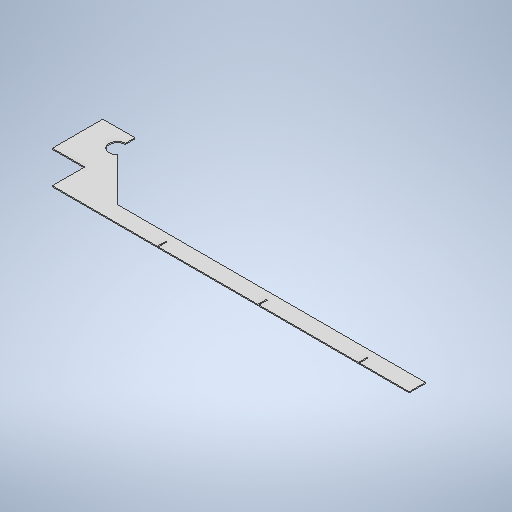
# Autodesk Inventor part: BSH 021 rib 1
Saved by Autodesk Inventor 2025 (Build 290162010, 162A)
## iProperties
Created: 2024-07-23
Part Number: BSH 021 rib 1
Material: 09g2s
Document SubType Name: Sheet Metal
Designer: admin
Density: 7.85 g/cm^3
Sheet Metal Rule: AISI304 3mm Die 32
Appearance: Default
Author: admin
Autodesk Inventor part; units mm, degrees
ref_plane "YZ Plane" through (0, 0, 0) normal (1, 0, 0) x (0, 1, 0)
ref_plane "XZ Plane" through (0, 0, 0) normal (0, 1, 0) x (-1, 0, 0)
ref_plane "XY Plane" through (0, 0, 0) normal (0, 0, 1) x (1, 0, 0)
sketch "Sketch1" plane through (0, 0, 0) normal (0, 0, 1) x (1, 0, 0)
  line L0 (1200, 2900) -> (-1200, 2900)
  line L1 (-1200, 2900) -> (-1200, 0)
  line L2 (-1200, 0) -> (1200, 0)
  line L3 (1200, 0) -> (1200, 2900)
  line L4 (1150, 2900) -> (1150, 0)
  line L5 (-1150, 0) -> (-1150, 2900) construction
  line L6 (0, 2900) -> (0, 50) construction
  line L7 (-1100, 200.463) -> (-949.537, 50)
  line L8 (-1200, 100) -> (-1100, 100)
  line L9 (-1100, 100) -> (-1100, 0)
  line L10 (-1100, 200.463) -> (-1150, 2900)
  arc A0 (-1100.463, 225.4587) -> (-1082.3223, 182.7853) centre (-1100, 200.463) ccw
  arc A1 (-1082.3223, 182.7853) -> (-1100.463, 225.4587) centre (-1100, 200.463) ccw construction
  line L11 (-1200, 255.463) -> (-1101.0187, 255.463)
  line L12 (0, 50) -> (-949.537, 50)
  line L13 (0, 50) -> (0, 0)
  line L14 (1504.8819, -225.894) -> (355.3449, -225.894)
  dimension "d3" = 2400
  dimension "d4" = 2900
  dimension "d5" = 50
  dimension "d6" = 100
  dimension "d7" = 50
  dimension "d8" = 2644.537
  dimension "d9" = 135
  dimension "d10" = 949.537
  dimension "d11" = 1149.537
  dimension "d12" = 136.061
  dimension "d13" = 50
  dimension "d14" = 100
  dimension "d15" = 212.7868
  dimension "d16" = 2700
  dimension "d17" = 55
  measures "d3" distance of L3.start L1.end
  measures "d4" distance of L1.end L1.start
  measures "d5" diameter of A0
  measures "d6" distance of L8.start L8.end
  measures "d7" distance between parallel lines of L1 L5
  measures "d8" distance between parallel lines of L0 L11
  measures "d9" angle of L12 L7
  measures "d10" distance of L6.end L7.end
  measures "d11" distance of L14.start L14.end
  measures "d12" angle of L7 L10
  measures "d13" distance between parallel lines of L2 L12
  measures "d14" distance from line of L1 L10.start
  measures "d15" distance of L10.start L7.end
  measures "d16" distance of L10.start L10.end
  measures "d17" vertical distance of L10.start L11.end
extrude "Plate1" add sketch "Sketch1" against normal blind 3 contours L10 A0 L7 L12 L13 L2 L9 L8 L1 L11
sketch "Sketch2" plane through (0, 0, 0) normal (0, 0, 1) x (1, 0, 0)
  line L0 (-1100, 0) -> (0, 0) projected
  line L1 (-156.6, 0) -> (-153.4, 0)
  line L2 (-153.4, 0) -> (-153.4, 26)
  line L3 (-153.4, 26) -> (-156.6, 26)
  line L4 (-156.6, 26) -> (-156.6, 0)
  point P0 (-155, 0)
  point P1 (-153.4, 0)
  dimension "d20" = 3.2
  dimension "d21" = 26
  dimension "d22" = 155
  constraints: 8 end point, 2 parallel, 1 horizontal, 1 horizontal alignment, 1 midpoint, 1 perpendicular, 1 point on line
  measures "d20" distance of L2.end L3.end
  measures "d21" distance of L3.end L1.start
  measures "d22" distance of L0.end point (-155, 0)
extrude "Extrusion1" cut sketch "Sketch2" against normal through all
pattern_linear "Rectangular Pattern1" count 3 spacing 310 along (-1, 0, 0) of "Extrusion1"
equation "\"d11\" = d10 + d18"
equation "\"d14\" = d6"
equation "\"d2\" = Thickness"
equation "\"BendReliefWidth\" = Thickness"
equation "\"BendReliefDepth\" = 0.5 * Thickness"
equation "\"CornerReliefSize\" = 4 * Thickness"
equation "\"MinimumRemnant\" = 2 * Thickness"
equation "\"TransitionRadius\" = BendRadius"
equation "\"JacobiRadiusSize\" = BendRadius"
equation "\"GapSize\" = Thickness"
equation "\"d18\" = d19"
equation "\"Thickness\" = 3"
equation "\"BendRadius\" = 5"
equation "\"d19\" = 200"
body "Solid1"
